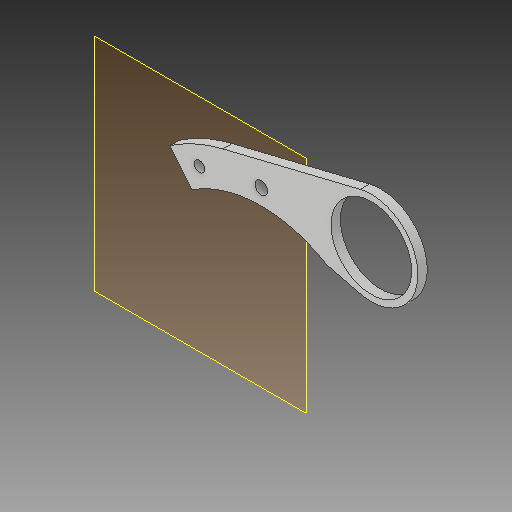
# Autodesk Inventor part: FrontMotorPlateB
Saved by Autodesk Inventor 2019.3 (Build 233278000, 278)
## iProperties
Created: 2019-05-08
Part Number: FrontMotorPlateB
Material: Generic
Document SubType Name: Modeling
Designer: eroldan
Density: 1 g/cm^3
Appearance: Default
Author: eroldan
Autodesk Inventor part; units mm, degrees
ref_plane "YZ Plane" through (0, 0, 0) normal (1, 0, 0) x (0, 1, 0)
ref_plane "XZ Plane" through (0, 0, 0) normal (0, 1, 0) x (-1, 0, 0)
ref_plane "XY Plane" through (0, 0, 0) normal (0, 0, 1) x (1, 0, 0)
ref_plane "Work Plane1" through (0, 0, 0) normal (0, 0, 1) x (1, 0, 0)
sketch "Sketch1" plane through (0, 0, 0) normal (0, 0, 1) x (1, 0, 0)
  circle A0 centre (91.7273, 29.791) radius 19.05 projected
  circle A1 centre (39.6359, 28.4758) radius 3 projected
  arc A2 (69.9962, 12.7276) -> (6.7276, 11.146) centre (39.6359, -39.0242) ccw
  arc A3 (69.9962, 12.7276) -> (71.0345, 12.3011) centre (72.0202, 16.1778) ccw projected
  line L0 (86.2932, 8.4211) -> (71.0345, 12.3011) projected
  arc A4 (86.2932, 8.4211) -> (86.4826, 51.2082) centre (91.7273, 29.791) ccw projected
  line L1 (21.44, 35.2803) -> (86.4826, 51.2082) projected
  arc A5 (21.44, 35.2803) -> (-3.5721, 24.1052) centre (39.6359, -39.0242) ccw
  line L2 (6.7276, 11.146) -> (-3.5721, 24.1052) projected
  circle A6 centre (10.4041, 22.5922) radius 2.5 projected
  point P0 (0, 0)
  constraints: 4 point on circle, 2 centre point, 2 point on line
extrude "Extrusion1" add sketch "Sketch1" along normal blind 4.4
body "Solid1"
